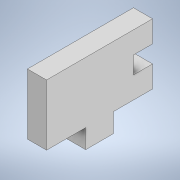
# Autodesk Inventor part: FondV2
Saved by Autodesk Inventor 2020 (Build 240168000, 168)
## iProperties
Created: 2019-11-07
Part Number: FondV2
Material: Générique
Document SubType Name: Modeling
Designer: erwan
Density: 1 g/cm^3
Appearance: Par défaut
Author: erwan
Autodesk Inventor part; units mm, degrees
ref_plane "YZ Plane" through (0, 0, 0) normal (1, 0, 0) x (0, 1, 0)
ref_plane "XZ Plane" through (0, 0, 0) normal (0, 1, 0) x (-1, 0, 0)
ref_plane "XY Plane" through (0, 0, 0) normal (0, 0, 1) x (1, 0, 0)
sketch "Esquisse1" plane through (0, 0, 0) normal (0, 1, 0) x (-1, 0, 0)
  line L0 (0, 0) -> (22, 0)
  line L1 (22, 0) -> (22, -122)
  line L2 (22, -122) -> (0, -122)
  line L3 (0, -122) -> (0, 0)
  dimension "d0" = 22
  dimension "d1" = 122
  constraints: 8 end point, 2 parallel, 1 horizontal, 1 perpendicular
  measures "d0" distance of L1.end L2.end
  measures "d1" distance of L0.end L1.end
extrude "Extrusion1" add sketch "Esquisse1" along normal blind 70
sketch "Esquisse2" plane through (0, 0, 0) normal (1, 0, 0) x (0, 0, -1)
  line L0 (0, 0) -> (45, 0)
  line L1 (122, 0) -> (0, 0) projected
  line L2 (45, 0) -> (45, -22)
  line L3 (45, -22) -> (77, -22)
  line L4 (77, -22) -> (77, 0)
  dimension "d4" = 45
  dimension "d5" = 22
  dimension "d6" = 32
  constraints: 8 end point, 3 perpendicular, 2 point on line
  measures "d4" distance of L0.start L0.end
  measures "d5" distance of L0.end L2.end
  measures "d6" distance of L2.end L3.end
extrude "Extrusion2" add sketch "Esquisse2" against normal blind 22
sketch "Esquisse3" plane through (0, 0, -122) normal (1, 0, 0) x (0, 0, -1)
  line L0 (-122, 70) -> (0, 70) projected
  line L1 (0, 70) -> (0, 45)
  line L2 (0, 0) -> (0, 70) projected
  line L3 (0, 45) -> (-22, 45)
  line L4 (-22, 45) -> (-22, 25)
  line L5 (-22, 25) -> (0, 25)
  point P0 (-122, 0)
  dimension "d9" = 25
  dimension "d10" = 22
  dimension "d11" = 20
  constraints: 8 end point, 3 perpendicular, 2 point on line
  measures "d9" distance of L0.end L1.end
  measures "d10" distance of L1.end L3.end
  measures "d11" distance of L3.end L4.end
extrude "Extrusion3" cut sketch "Esquisse3" against normal blind 22
